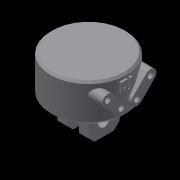
# Autodesk Inventor part: VacuumTubeHolderBase
Saved by Autodesk Inventor 2015 SP1 (Build 190203100, 203)
## iProperties
Created: 2015-06-28
Part Number: VacuumTubeHolderBase
Material: Generic
Document SubType Name: Modeling
Designer: Val
Density: 1 g/cm^3
Appearance: Default
Author: Val
Autodesk Inventor part; units mm, degrees
sketch "Base" plane through (0, 0, 0) normal (0, 0, 1) x (1, 0, 0)
  circle A0 centre (0, 0) radius 19.5
  dimension "d0" = 39
  constraints: 1 centre point, 1 coincident
  measures "d0" diameter of A0
extrude "BaseFeature" add sketch "Base" along normal blind 20
sketch "Mount" plane through (0, 0, 0) normal (0, 0, -1) x (-1, 0, 0)
  line L0 (8, 8) -> (-8, 8) construction
  line L1 (-8, 8) -> (-8, -8) construction
  line L2 (-8, -8) -> (8, -8) construction
  line L3 (8, -8) -> (8, 8) construction
  line L4 (27.3, 0) -> (-27.3, 0) construction
  line L5 (0, -27.3) -> (0, 27.3) construction
  line L6 (8, 8) -> (3, 8)
  line L7 (3, 8) -> (3, -8)
  line L8 (3, -8) -> (8, -8)
  line L9 (8, -8) -> (8, 8)
  line L10 (-8, 8) -> (-3, 8)
  line L11 (-3, 8) -> (-3, -8)
  line L12 (-3, -8) -> (-8, -8)
  line L13 (-8, -8) -> (-8, 8)
  point P0 (0, 0)
  point P1 (8, 0)
  point P2 (0, -8)
  dimension "d3" = 16
  dimension "d4" = 16
  dimension "d5" = 6
  constraints: 24 end point, 6 parallel, 4 point on line, 3 horizontal, 3 perpendicular, 2 midpoint, 1 collinear
  measures "d3" distance of L1.end L2.end
  measures "d4" distance of L2.end L0.start
  measures "d5" distance between parallel lines of L11 L7
extrude "MountFeature" add sketch "Mount" along normal blind 14
chamfer "MountChamferFeature" distance 3 angle 45 4 edges at (-5.5, -8, -14) (5.5, -8, -14) (5.5, 8, -14) (-5.5, 8, -14)
chamfer "BaseChamferBottomFeature" distance 2 angle 45 1 edges at (-19.5, 0, 0)
chamfer "BaseChamferTopFeature" distance 1 angle 45 1 edges at (-19.5, 0, 20)
sketch "Sketch4" plane through (-8, -8, 0) normal (-1, 0, 0) x (0, 0, 1)
  line L0 (-14, 13) -> (-14, 3) construction
  line L1 (-14, 8) -> (0, 8) construction
  line L2 (0, 16) -> (0, 0) construction
  circle A0 centre (-7, 8) radius 3
  dimension "d20" = 6
  constraints: 3 midpoint, 2 end point, 1 centre point
  measures "d20" diameter of A0
hole "MountHoleFeature" at (-8, 0, -7) direction (1, 0, 0) diameter 6 end through all
ref_plane "SurfaceMountsPlane" through (8, 8, 0) normal (1, 0, 0) x (0, 0, -1)
sketch "SurfaceMounts" plane through (8, 8, 0) normal (1, 0, 0) x (0, 0, -1)
  circle A0 centre (-7, -12) radius 1.5
  circle A1 centre (-14, -19) radius 1.5
  line L0 (-12.9393, -20.0607) -> (-5.9393, -13.0607)
  line L1 (-15.0607, -17.9393) -> (-8.0607, -10.9393)
  line L2 (-2, -27.5) -> (-2, 11.5) construction
  circle A2 centre (-14, -19) radius 3
  circle A3 centre (-7, -12) radius 3
  line L3 (-16.1213, -16.8787) -> (-9.1213, -9.8787)
  line L4 (-2, -27.5) -> (-19, -27.5) construction
  line L5 (-11.8787, -21.1213) -> (-4.8787, -14.1213)
  line L6 (-19, 11.5) -> (-19, -27.5) construction
  line L7 (-19, -8) -> (-2, -8) construction
  circle A4 centre (-7, -4) radius 1.5
  circle A5 centre (-14, 3) radius 1.5
  line L8 (-12.9393, 4.0607) -> (-5.9393, -2.9393)
  line L9 (-15.0607, 1.9393) -> (-8.0607, -5.0607)
  circle A6 centre (-14, 3) radius 3
  circle A7 centre (-7, -4) radius 3
  line L10 (-16.1213, 0.8787) -> (-9.1213, -6.1213)
  line L11 (-11.8787, 5.1213) -> (-4.8787, -1.8787)
  dimension "d29" = 3
  dimension "d30" = 45
  dimension "d31" = 6
  dimension "d32" = 6
  dimension "d33" = 8.5
  dimension "d34" = 5
  dimension "d35" = 5
  dimension "d36" = 4
  dimension "d55" = 8.5
  constraints: 18 end point, 16 point on circle, 12 symmetric about line, 8 centre point, 8 tangent, 4 coincident, 2 midpoint, 1 equal radius, 1 perpendicular, 4 other
  measures "d29" diameter of A0
  measures "d30" angle of L2 L0
  measures "d31" diameter of A2
  measures "d32" diameter of A3
  measures "d33" distance from line of A1.centre L4
  measures "d34" distance from line of L6 A1.centre
  measures "d35" distance from line of L2 A0.centre
  measures "d36" distance from line of L7 A0.centre
  measures "d55" vertical distance of L6.start A6.centre
extrude "SurfaceMountsFeature" add sketch "SurfaceMounts" along normal blind 13 contours A0 L1 A3 L0 | A0 L0 A3 L1 | A3 L0 A2 L1 | L1 A2 L3 A3 | A3 L5 A2 L0 | A2 L0 A1 L1 | L1 A1 L0 A2 | A4 L8 A7 L9 | A4 L9 A7 L8 | A7 L9 A6 L8 | L8 A6 L11 A7 | A7 L10 A6 L9 | A6 L9 A5 L8 | L8 A5 L9 A6
ref_plane "VentHolesPlane" through (8, -8, 0) normal (0.5, 0.866, 0) x (0, 0, -1)
sketch "FixHoles" plane through (21, 8, 0) normal (1, 0, 0) x (0, -1, 0)
  circle A0 centre (19, -14) radius 1.5 projected
  circle A1 centre (12, -7) radius 1.5 projected
  circle A2 centre (4, -7) radius 1.5 projected
  circle A3 centre (-3, -14) radius 1.5 projected
  point P0 (8, 0)
hole "FixHolesFeature" at (21, -4, 7) at (21, -11, 14) at (21, 4, 7) at (21, 11, 14) direction (-1, 0, 0) diameter 3 depth 9 tip angle 118
ref_plane "VentHolesOffsetPlane" through (23, 17.9808, 0) normal (0.5, 0.866, 0) x (0, 0, -1)
sketch "VentHoles" plane through (23, 17.9808, 0) normal (0.5, 0.866, 0) x (0, 0, -1)
  line L0 (-5.5, 11.937) -> (-15.5, 14.5642) construction
  circle A0 centre (-5.5, 11.937) radius 1
  circle A1 centre (-15.5, 14.5642) radius 1
  line L1 (-5.7541, 10.9699) -> (-15.7541, 13.597)
  line L2 (-5.2459, 12.9042) -> (-15.2459, 15.5313)
  line L3 (-2, -8.5718) -> (-2, 30.4282) construction
  line L4 (-5.5, 7.937) -> (-15.5, 10.5642) construction
  circle A2 centre (-5.5, 7.937) radius 1
  circle A3 centre (-15.5, 10.5642) radius 1
  line L5 (-5.7541, 6.9699) -> (-15.7541, 9.597)
  line L6 (-5.2459, 8.9042) -> (-15.2459, 11.5313)
  line L7 (-2, -8.5718) -> (-2, 30.4282) projected
  line L8 (-19, 30.4282) -> (-19, -8.5718) construction
  point P0 (-11.8787, 4.9964)
  dimension "d57" = 2
  dimension "d61" = 10
  dimension "d67" = 4
  dimension "d81" = 3.5
  dimension "d82" = 3.5
  dimension "d83" = 2.9406
  dimension "d84" = 75.28
  constraints: 14 end point, 8 point on circle, 4 centre point, 4 coincident, 4 tangent, 1 collinear, 1 equal radius, 1 vertical, 13 other
  measures "d57" diameter of A0
  measures "d61" horizontal distance of L0.start L0.end
  measures "d67" distance of A0.centre A2.centre
  measures "d81" distance from line of A2.centre L3
  measures "d82" distance from line of L8 A3.centre
  measures "d83" vertical distance of A2.centre point (-11.879, 4.996)
  measures "d84" angle of L6 L7
extrude "VentHolesFeature" cut sketch "VentHoles" against normal blind 14
ref_plane "LogoPlane" through (19, 8, 0) normal (1, 0, 0) x (0, 0, -1)
sketch "Logo" plane through (19, 8, 0) normal (1, 0, 0) x (0, 0, -1)
  line L0 (-12.8455, -6.5425) -> (-12.8455, -5.3425)
  line L1 (-17.3455, -6.5425) -> (-12.8455, -6.5425)
  line L2 (-12.2455, -4.7425) -> (-17.9455, -4.7425)
  line L3 (-12.8455, -5.3425) -> (-17.3455, -5.3425)
  line L4 (-12.8455, -11.0425) -> (-12.2455, -11.0425)
  line L5 (-12.8455, -11.0425) -> (-12.8455, -11.6425)
  line L6 (-17.3455, -5.3425) -> (-17.3455, -6.5425)
  line L7 (-17.3455, -7.7425) -> (-12.8455, -7.7425)
  line L8 (-14.0455, -9.8425) -> (-14.0455, -8.9425)
  line L9 (-16.1455, -9.8425) -> (-14.0455, -9.8425)
  line L10 (-16.1455, -8.9425) -> (-16.1455, -9.8425)
  line L11 (-12.2455, -11.0425) -> (-12.2455, -4.7425)
  line L12 (-17.9455, -4.7425) -> (-17.9455, -11.6425)
  line L13 (-12.8455, -7.7425) -> (-12.8455, -11.0425)
  line L14 (-17.3455, -11.0425) -> (-17.3455, -7.7425)
  line L15 (-17.9455, -11.6425) -> (-12.8455, -11.6425)
  line L16 (-14.0455, -8.9425) -> (-16.1455, -8.9425)
  line L17 (-12.8455, -11.0425) -> (-17.3455, -11.0425)
  circle A0 centre (-14, -19) radius 1.5
  circle A1 centre (-14, 3) radius 1.5
  point P0 (0, -8)
  dimension "d101" = 90
  dimension "d102" = 90
  dimension "d103" = 90
  dimension "d104" = 90
  dimension "d105" = 0.6
  dimension "d106" = 1.8
  dimension "d107" = 3.9
  dimension "d108" = 5.1
  dimension "d109" = 5.7
  dimension "d110" = 0.6
  dimension "d111" = 1.8
  dimension "d112" = 3
  dimension "d113" = 4.2
  dimension "d114" = 5.1
  dimension "d115" = 6.3
  dimension "d116" = 6.9
  dimension "d117" = 12.2455
  dimension "d118" = 3.0425
  dimension "d119" = 12.8455
  dimension "d120" = 17.3455
  constraints: 36 end point, 12 parallel, 2 centre point, 1 horizontal, 1 vertical
  measures "d101" angle of L11 L4
  measures "d102" angle of L4 L13
  measures "d103" angle of L4 L5
  measures "d104" angle of L4 L14
  measures "d105" distance between parallel lines of L11 L0
  measures "d106" distance between parallel lines of L11 L8
  measures "d107" distance between parallel lines of L11 L10
  measures "d108" distance between parallel lines of L11 L6
  measures "d109" distance between parallel lines of L11 L12
  measures "d110" distance between parallel lines of L2 L3
  measures "d111" distance between parallel lines of L2 L1
  measures "d112" distance between parallel lines of L2 L7
  measures "d113" distance between parallel lines of L2 L16
  measures "d114" distance between parallel lines of L2 L9
  measures "d115" distance between parallel lines of L2 L17
  measures "d116" distance between parallel lines of L2 L15
  measures "d117" distance from line of point (0, -8) L11
  measures "d118" distance from line of point (0, -8) L4
  measures "d119" distance from line of point (0, -8) L13
  measures "d120" distance from line of point (0, -8) L14
extrude "LogoPositiveFeature" add sketch "Logo" along normal blind 1 contours L1 L6 L3 L0 | L17 L14 L7 L13
extrude "LogoNegativeFeature" cut sketch "Logo" along normal blind 5 contours L11 L4 L5 L15 L12 L2
equation "\"d55\" = d33"
equation "\"d82\" = d81"
